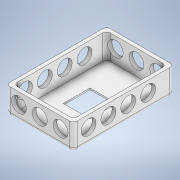
# Autodesk Inventor part: TopCover
Saved by Autodesk Inventor 2021 (Build 250183000, 183)
## iProperties
Created: 2022-12-30
Part Number: TopCover
Material: ABS Plastic
Document SubType Name: Modeling
Designer: Nihal
Density: 1.06 g/cm^3
Appearance: Smooth - White
Author: Nihal
Autodesk Inventor part; units mm, degrees
ref_plane "YZ Plane" through (0, 0, 0) normal (1, 0, 0) x (0, 1, 0)
ref_plane "XZ Plane" through (0, 0, 0) normal (0, 1, 0) x (-1, 0, 0)
ref_plane "XY Plane" through (0, 0, 0) normal (0, 0, 1) x (1, 0, 0)
sketch "Sketch1" plane through (0, 0, 0) normal (0, 1, 0) x (-1, 0, 0)
  line L0 (33.92, 50.615) -> (-33.92, 50.615)
  line L1 (-33.92, 50.615) -> (-33.92, -50.615)
  line L2 (-33.92, -50.615) -> (33.92, -50.615)
  line L3 (33.92, -50.615) -> (33.92, 50.615)
  line L4 (33.92, 50.615) -> (-33.92, -50.615) construction
  line L5 (-33.92, 50.615) -> (33.92, -50.615) construction
  point P0 (0, 0)
  dimension "d0" = 67.84
  dimension "d1" = 101.23
  constraints: 12 end point, 2 midpoint, 2 parallel, 1 horizontal, 1 perpendicular
  measures "d0" distance of L2.end L1.end
  measures "d1" distance of L2.end L0.start
extrude "Extrusion1" add sketch "Sketch1" along normal blind 26.5
fillet "Fillet1" radius 4 8 edges at (33.92, 13.25, 50.615) (33.92, 0, 0) (33.92, 13.25, -50.615) (-33.92, 13.25, -50.615) (0, 0, -50.615) (0, 0, 50.615) (-33.92, 13.25, 50.615) (-33.92, 0, 0)
sketch "Sketch2" plane through (0, 26.5, 0) normal (0, 1, 0) x (1, 0, 0)
  line L0 (30.2, 46.895) -> (-30.2, 46.895)
  line L1 (-30.2, 46.895) -> (-30.2, -46.895)
  line L2 (-30.2, -46.895) -> (30.2, -46.895)
  line L3 (30.2, -46.895) -> (30.2, 46.895)
  line L4 (30.2, 46.895) -> (-30.2, -46.895) construction
  line L5 (-30.2, 46.895) -> (30.2, -46.895) construction
  line L6 (-29.92, -50.615) -> (29.92, -50.615) projected
  line L7 (33.92, -46.615) -> (33.92, 46.615) projected
  point P0 (0, 0)
  dimension "d5" = 3.72
  dimension "d6" = 3.72
  constraints: 12 end point, 2 midpoint, 2 parallel, 1 horizontal, 1 perpendicular
  measures "d5" distance between parallel lines of L6 L2
  measures "d6" distance between parallel lines of L7 L3
extrude "Extrusion2" cut sketch "Sketch2" against normal blind 25
fillet "Fillet2" radius 4 4 edges at (30.2, 14, -46.895) (30.2, 14, 46.895) (-30.2, 14, -46.895) (-30.2, 14, 46.895)
sketch "Sketch3" plane through (0, 0, 0) normal (0, -1, 0) x (1, 0, 0)
  line L0 (-13.5, -13.5) -> (13.5, -13.5)
  line L1 (13.5, -13.5) -> (13.5, 13.5)
  line L2 (13.5, 13.5) -> (-13.5, 13.5)
  line L3 (-13.5, 13.5) -> (-13.5, -13.5)
  line L4 (-13.5, -13.5) -> (13.5, 13.5) construction
  line L5 (13.5, -13.5) -> (-13.5, 13.5) construction
  point P0 (0, 0)
  dimension "d10" = 27
  dimension "d11" = 27
  constraints: 12 end point, 2 midpoint, 2 parallel, 1 horizontal, 1 perpendicular
  measures "d10" distance of L2.end L1.end
  measures "d11" distance of L1.end L0.end
extrude "Extrusion4" cut sketch "Sketch3" against normal through all
sketch "Sketch4" plane through (-33.92, 4, 46.615) normal (-1, 0, 0) x (0, 0, 1)
  circle A0 centre (-11.226, 11.5) radius 7.5
  circle A1 centre (-31.226, 11.5) radius 7.5
  circle A2 centre (-51.226, 11.5) radius 7.5
  circle A3 centre (-71.226, 11.5) radius 7.5
  line L0 (0, 22.5) -> (0, 0) projected
  line L1 (-93.23, 22.5) -> (0, 22.5) projected
  point P0 (-46.615, -4)
  dimension "d17" = 15
  dimension "d18" = 15
  dimension "d19" = 20
  dimension "d20" = 15
  dimension "d21" = 15
  dimension "d22" = 20
  dimension "d23" = 20
  dimension "d24" = 11.226
  dimension "d25" = 11
  dimension "d26" = 11
  dimension "d27" = 11
  dimension "d28" = 11
  constraints: 4 centre point
  measures "d17" diameter of A0
  measures "d18" diameter of A1
  measures "d19" distance of A1.centre A0.centre
  measures "d20" diameter of A2
  measures "d21" diameter of A3
  measures "d22" distance of A2.centre A1.centre
  measures "d23" distance of A3.centre A2.centre
  measures "d24" distance from line of L0 A0.centre
  measures "d25" distance from line of L1 A0.centre
  measures "d26" distance from line of L1 A1.centre
  measures "d27" distance from line of L1 A2.centre
  measures "d28" distance from line of L1 A3.centre
extrude "Extrusion5" cut sketch "Sketch4" against normal through all
sketch "Sketch5" plane through (29.92, 4, -50.615) normal (0, 0, -1) x (-1, 0, 0)
  line L0 (59.84, 22.5) -> (59.84, 0) projected
  line L1 (0, 22.5) -> (59.84, 22.5) projected
  line L2 (59.84, 0) -> (0, 22.5) construction
  line L3 (59.84, 0) -> (0, 0) projected
  line L4 (59.84, 22.5) -> (0, 0) construction
  circle A0 centre (29.92, 11.25) radius 7.5
  circle A1 centre (50.92, 11.25) radius 7.5
  circle A2 centre (8.92, 11.25) radius 7.5
  line L5 (0, 0) -> (0, 22.5) projected
  point P0 (29.92, -4)
  dimension "d31" = 15
  dimension "d32" = 15
  dimension "d33" = 15
  dimension "d34" = 21
  dimension "d35" = 21
  dimension "d36" = 8.92
  dimension "d37" = 8.92
  constraints: 4 end point, 3 centre point, 1 midpoint
  measures "d31" diameter of A0
  measures "d32" diameter of A1
  measures "d33" diameter of A2
  measures "d34" distance of A0.centre A1.centre
  measures "d35" distance of A2.centre A0.centre
  measures "d36" distance from line of L0 A1.centre
  measures "d37" distance from line of L5 A2.centre
extrude "Extrusion6" cut sketch "Sketch5" against normal through all contours A0 | A1 | A2
body "Solid1"
